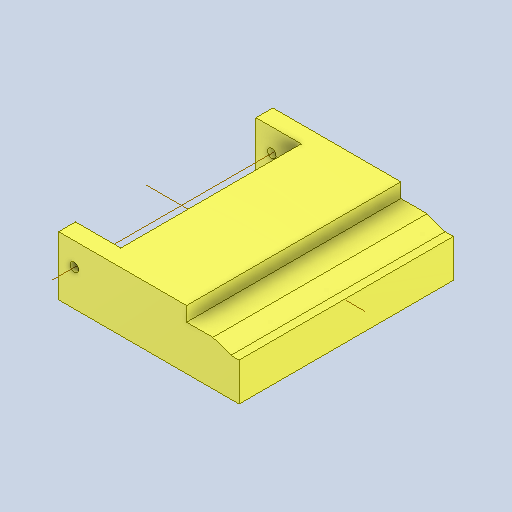
# Autodesk Inventor part: Type 1A R6主滑台:1
Saved by Autodesk Inventor 2025 (Build 290162000, 162)
## iProperties
Created: 2024-09-22
Part Number: Type 1A R6主滑台:1
Material: 密度7850的鋼
Document SubType Name: Modeling
Designer: veter
Density: 7.84999 g/cm^3
Appearance: 平滑 - 黃色
Mass: 358314 g
Surface Area: 10286.9 cm^2
Volume: 45645.1 cm^3
Stock Number: 6
Author: veter
Autodesk Inventor part; units mm, degrees
ref_plane "YZ Plane" through (0, 0, 0) normal (1, 0, 0) x (0, 1, 0)
ref_plane "XZ Plane" through (0, 0, 0) normal (0, 1, 0) x (-1, 0, 0)
ref_plane "XY Plane" through (0, 0, 0) normal (0, 0, 1) x (1, 0, 0)
sketch "草圖1" plane through (0, 0, 0) normal (0, 0, 1) x (0, 1, 0)
  line L0 (-110, 48) -> (70, 48)
  line L1 (70, 48) -> (70, -502)
  line L2 (70, -502) -> (-110, -502)
  line L3 (-110, -502) -> (-110, 48)
  line L4 (70, -342) -> (26, -342)
  line L5 (26, -342) -> (26, -422)
  line L6 (26, -422) -> (6, -476.9495)
  line L7 (6, -476.9495) -> (6, -502)
  point P0 (0, 0)
  dimension "d0" = 110
  dimension "d1" = 48
  dimension "d2" = 180
  dimension "d3" = 550
  dimension "d10" = 136
  dimension "d11" = 20
  dimension "d12" = 20
  dimension "d13" = 80
  dimension "d19" = 160
  constraints: 16 end point, 3 parallel, 3 perpendicular, 2 point on line, 1 horizontal
  measures "d0" distance from line of L3 point (0, 0)
  measures "d1" distance from line of L0 point (0, 0)
  measures "d2" distance of L0.start L0.end
  measures "d3" distance of L2.end L0.start
  measures "d10" distance between parallel lines of L3 L5
  measures "d11" distance between parallel lines of L5 L7
  measures "d12" angle of L6 L7
  measures "d13" distance of L4.end L5.end
  measures "d19" distance between parallel lines of L2 L4
extrude "擠出1" add sketch "草圖1" along normal mid plane 653 contours L0 L1 L4 L5 L6 L7 L2 L3
sketch "草圖2" plane through (0, 0, 0) normal (0, 0, 1) x (0, 1, 0)
  line L0 (70, -90) -> (-110, -90)
  line L1 (-110, 48) -> (70, 48) projected
  line L2 (70, 48) -> (70, -342) projected
  line L3 (6, -502) -> (-110, -502) projected
  line L4 (-110, -502) -> (-110, 48) projected
  line L5 (70, -103.9214) -> (70, -178.9214)
  line L6 (70, -342) -> (26, -342) projected
  line L7 (26, -342) -> (26, -422) projected
  line L8 (26, -422) -> (6, -476.9495) projected
  line L9 (6, -476.9495) -> (6, -502) projected
  point P0 (0, 0)
  dimension "d6" = 90
  constraints: 4 end point, 2 point on line, 1 collinear, 1 horizontal, 1 vertical
  measures "d6" distance from line of L0 point (0, 0)
extrude "擠出2" cut sketch "草圖2" along normal mid plane 550 contours L0 L4 L1 L2
sketch "草圖3" plane through (0, 0, 0) normal (0, 0, 1) x (0, 1, 0)
  circle A0 centre (0, 0) radius 13.25
  dimension "d4" = 653
  dimension "d14" = 26.5
  constraints: 1 centre point, 1 coincident
  measures "d14" diameter of A0
extrude "擠出3" cut sketch "草圖3" along normal through all both and the other way through all
equation "\"d7\" = Width"
equation "\"th6\" = T1A_th6"
equation "\"Width\" = T1A_R6_Width"
equation "\"T1A_th6\" = 45deg"
equation "\"T1A_R1\" = 585.5331"
equation "\"T1A_R3\" = 252.3048"
equation "\"T1A_R4\" = 320.6953"
equation "\"T1A_R5\" = 419.3047"
equation "\"T1A_R7\" = -221.7475"
equation "\"T1A_R8\" = 369.2781"
equation "\"T1A_R1_Width\" = 756"
equation "\"T1A_R2_Width\" = 756"
equation "\"T1A_R3_Width\" = 344"
equation "\"T1A_R4_Width\" = 756"
equation "\"T1A_Joint_Width\" = 756"
equation "\"T1A_R6_Width\" = 550"
